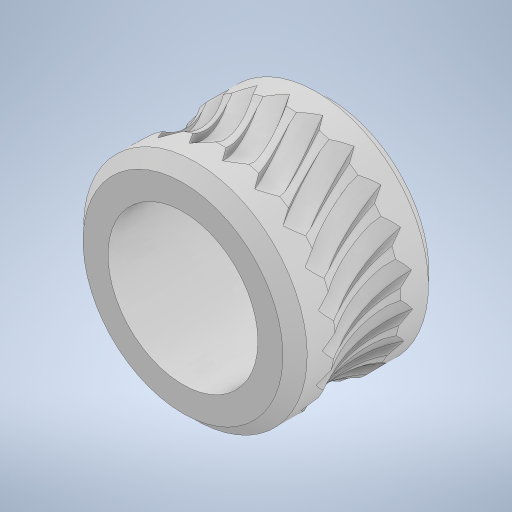
# Autodesk Inventor part: engranatge_final_3
Saved by Autodesk Inventor 2024.2 (Build 282272000, 272)
## iProperties
Created: 2024-03-04
Part Number: engranatge_final_3
Material: Genérico
Document SubType Name: Modeling
Designer: riera
Density: 1 g/cm^3
Appearance: Valor por defecto
Author: riera
Autodesk Inventor part; units mm, degrees
ref_plane "YZ Plane" through (0, 0, 0) normal (1, 0, 0) x (0, 1, 0)
ref_plane "XZ Plane" through (0, 0, 0) normal (0, 1, 0) x (-1, 0, 0)
ref_plane "pla dent" through (0, 0, 0) normal (0.4472128, 0, 0.8944276) x (0, 1, 0)
sketch "Boceto2" plane through (0, 0, 0) normal (1, 0, 0) x (0, 1, 0)
  line L0 (0, 21.915) -> (30, 21.915)
  line L1 (30, -21.915) -> (0, -21.915)
  line L2 (0, -21.915) -> (0, 21.915)
  arc A0 (33.5581, 9.9015) -> (33.5581, -9.9015) centre (50.9351, 0) ccw
  line L3 (50.9351, 0) -> (88.1071, 0) construction
  line L4 (33.5581, 18.1903) -> (30, 21.915)
  line L5 (33.5581, -18.1903) -> (30, -21.915)
  line L6 (33.5581, 18.1903) -> (33.5581, 9.9015)
  line L7 (33.5581, -9.9015) -> (33.5581, -18.1903)
  point P0 (0, 0)
  point P1 (82.623, 0)
  point P2 (0, 0)
  dimension "d1" = 43.83
  dimension "d3" = 40
  dimension "d30" = 30
  dimension "d32" = 136.31
  dimension "d33" = 3.5581
  constraints: 16 end point, 3 parallel, 2 horizontal, 2 horizontal alignment, 2 perpendicular, 2 point on circle, 2 symmetric about line, 1 centre point, 1 midpoint
  measures "d1" distance of L1.end L0.start
  measures "d3" diameter of A0
  measures "d30" distance of L0.start L0.end
  measures "d32" angle of L6 L4
  measures "d33" horizontal distance of L4.start L0.end
revolve "Revolución1" add sketch "Boceto2" angle 360 about axis through (0, 0, -21.915) along (0, 0, 1)
sketch "Boceto3" plane through (0, 0, 21.915) normal (0, 0, 1) x (1, 0, 0)
  circle A0 centre (0, 0) radius 75
  dimension "d8" = 150
  constraints: 1 centre point, 1 coincident
  measures "d8" diameter of A0
surface extrude "diametre separacio" sketch "Boceto3" against normal blind 43.835 shown no curves A0
sketch "Boceto4" plane through (0, 0, 0) normal (0.4472128, 0, 0.8944276) x (0, 1, 0)
  line L0 (60, -6.8358) -> (60, 6.8358)
  line L1 (60, 6.8358) -> (40.835, 6.8358)
  line L2 (40.835, 6.8358) -> (30, 2.8921)
  line L3 (30, 2.8921) -> (30, -2.8921)
  line L4 (30, -2.8921) -> (40.835, -6.8358)
  line L5 (60, -6.8358) -> (40.835, -6.8358)
  line L6 (35, 0) -> (35, -4.712) construction
  point P0 (0, 0)
  point P1 (60, 0)
  point P2 (60, 0)
  point P3 (30, 0)
  dimension "d11" = 60
  dimension "d16" = 20
  dimension "d17" = 19.165
  dimension "d18" = 30
  dimension "d19" = 25
  dimension "d20" = 4.712
  constraints: 14 end point, 3 horizontal alignment, 2 midpoint, 2 parallel, 2 vertical, 1 coincident, 1 horizontal, 1 perpendicular, 1 point on line
  measures "d11" distance of point (0, 0) point (60, 0)
  measures "d16" angle of L4 L5
  measures "d17" distance of L0.start L4.end
  measures "d18" distance between parallel lines of L3 L0
  measures "d19" distance from line of L6.start L0
  measures "d20" distance of L6.end L6.start
revolve "Revolución2" cut sketch "Boceto4" angle 360 about axis through (6.1141, 60, -3.057) along (-0.8944276, 0, 0.4472128)
pattern_circular "Patrón circular1" count 21 over 360 about axis through (0, 0, -10) along (0, 0, 1) of "Revolución2"
sketch "Boceto5" plane through (0, 0, 21.915) normal (0, 0, 1) x (1, 0, 0)
  circle A0 centre (0, 0) radius 22.5
  dimension "d25" = 45
  constraints: 1 centre point, 1 coincident
  measures "d25" diameter of A0
extrude "Extrusión1" cut sketch "Boceto5" against normal blind 43.835
